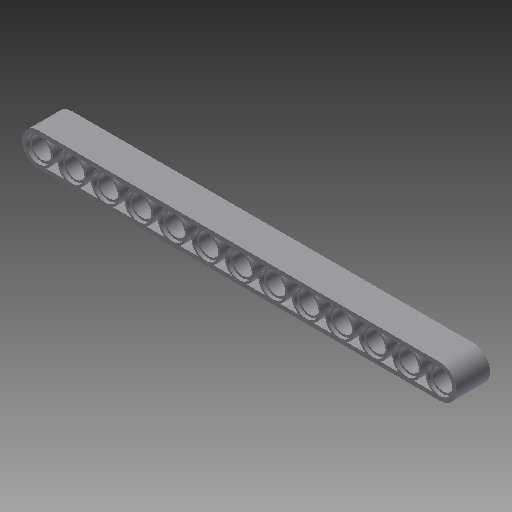
# Autodesk Inventor part: 13M Beam
Saved by Autodesk Inventor 2018 (Build 220112000, 112)
## iProperties
Created: 2014-02-10
Part Number: 13M Beam
Document SubType Name: Modeling
Designer: jleonard
Density: 1 g/cm^3
Material: Generic
Appearance: Default
Author: jleonard
Autodesk Inventor part; units mm, degrees
ref_plane "YZ Plane" through (0, 0, 0) normal (1, 0, 0) x (0, 1, 0)
ref_plane "XZ Plane" through (0, 0, 0) normal (0, 1, 0) x (-1, 0, 0)
ref_plane "XY Plane" through (0, 0, 0) normal (0, 0, 1) x (1, 0, 0)
sketch "Sketch2" plane through (0, 0, 0) normal (0, 0, 1) x (1, 0, 0)
  arc A0 (-48, 4) -> (-48, -4) centre (-48, 0) ccw
  arc A1 (48, -4) -> (48, 4) centre (48, 0) ccw
  line L0 (-48, 4) -> (48, 4)
  line L1 (-48, -4) -> (48, -4)
  line L2 (-72.8, 0) -> (72.8, 0) projected
  line L3 (0, -5.6) -> (0, 5.6) projected
  point P0 (0, 0)
  dimension "d0" = 4
  dimension "d1" = 4
  dimension "d2" = 96
  dimension "d3" = 0
  dimension "d4" = 48
  dimension "d9" = 180
  dimension "d10" = 0
  dimension "d225" = 96
  constraints: 6 point on circle, 4 end point, 2 centre point, 2 point on line, 2 tangent
  measures "d0" radius of A0
  measures "d1" radius of A1
  measures "d2" distance of A1.centre A0.centre
  measures "d3" distance from line of A0.centre L2
  measures "d4" distance from line of A0.centre L3
  measures "d9" angle of L0 L2
  measures "d10" distance from line of L2 A1.centre
  measures "d225" distance of L1.start L1.end
extrude "Extrusion1" add sketch "Sketch2" along normal blind 8
sketch "Sketch23" plane through (0, 0, 8) normal (0, 0, 1) x (1, 0, 0)
  arc A0 (-48, 4) -> (-48, -4) centre (-48, 0) ccw projected
  circle A1 centre (-48, 0) radius 2.5
  line L0 (-72.8, 0) -> (72.8, 0) projected
  circle A2 centre (-40, 0) radius 2.5
  circle A3 centre (-32, 0) radius 2.5
  circle A4 centre (-24, 0) radius 2.5
  circle A5 centre (-16, 0) radius 2.5
  circle A6 centre (-8, 0) radius 2.5
  circle A7 centre (0, 0) radius 2.5
  circle A8 centre (8, 0) radius 2.5
  circle A9 centre (16, 0) radius 2.5
  circle A10 centre (24, 0) radius 2.5
  circle A11 centre (32, 0) radius 2.5
  circle A12 centre (40, 0) radius 2.5
  circle A13 centre (48, 0) radius 2.5
  dimension "d226" = 5
  dimension "d232" = 8
  constraints: 13 centre point, 1 coincident, 1 horizontal, 24 other
  measures "d226" diameter of A1
  measures "d232" distance of A1.centre A2.centre
extrude "Extrusion22" cut sketch "Sketch23" against normal through all
sketch "Sketch24" plane through (0, 0, 8) normal (0, 0, 1) x (1, 0, 0)
  circle A0 centre (48, 0) radius 2.5 projected
  circle A1 centre (40, 0) radius 2.5 projected
  circle A2 centre (32, 0) radius 2.5 projected
  circle A3 centre (24, 0) radius 2.5 projected
  circle A4 centre (16, 0) radius 2.5 projected
  circle A5 centre (8, 0) radius 2.5 projected
  circle A6 centre (0, 0) radius 2.5 projected
  circle A7 centre (-8, 0) radius 2.5 projected
  circle A8 centre (-16, 0) radius 2.5 projected
  circle A9 centre (-24, 0) radius 2.5 projected
  circle A10 centre (-32, 0) radius 2.5 projected
  circle A11 centre (-40, 0) radius 2.5 projected
  circle A12 centre (-48, 0) radius 2.5 projected
  arc A13 (-48, 4) -> (-48, -4) centre (-48, 0) ccw projected
  circle A14 centre (-48, 0) radius 3
  line L0 (-72.8, 0) -> (72.8, 0) projected
  circle A15 centre (-40, 0) radius 3
  circle A16 centre (-32, 0) radius 3
  circle A17 centre (-24, 0) radius 3
  circle A18 centre (-16, 0) radius 3
  circle A19 centre (-8, 0) radius 3
  circle A20 centre (0, 0) radius 3
  circle A21 centre (8, 0) radius 3
  circle A22 centre (16, 0) radius 3
  circle A23 centre (24, 0) radius 3
  circle A24 centre (32, 0) radius 3
  circle A25 centre (40, 0) radius 3
  circle A26 centre (48, 0) radius 3
  dimension "d236" = 6
  dimension "d242" = 8
  constraints: 13 centre point, 1 coincident, 1 horizontal, 24 other
  measures "d236" diameter of A14
  measures "d242" distance of A14.centre A15.centre
extrude "Extrusion23" cut sketch "Sketch24" against normal blind 0.8 contours L0 A26 A0 | A0 L0 A26 | A14 L0 A12 | L0 A12 A14 | A15 L0 A11 | L0 A11 A15 | A16 L0 A10 | L0 A10 A16 | A17 L0 A9 | L0 A9 A17 | A18 L0 A8 | L0 A8 A18 | A19 L0 A7 | L0 A7 A19 | A20 L0 A6 | L0 A6 A20 | A21 L0 A5 | L0 A5 A21 | A22 L0 A4 | L0 A4 A22 | A23 L0 A3 | L0 A3 A23 | A24 L0 A2 | L0 A2 A24 | A25 L0 A1 | L0 A1 A25
sketch "Sketch25" plane through (0, 0, 0) normal (0, 0, -1) x (-1, 0, 0)
  circle A0 centre (-48, 0) radius 2.5 projected
  circle A1 centre (-40, 0) radius 2.5 projected
  circle A2 centre (-32, 0) radius 2.5 projected
  circle A3 centre (-24, 0) radius 2.5 projected
  circle A4 centre (-16, 0) radius 2.5 projected
  circle A5 centre (-8, 0) radius 2.5 projected
  circle A6 centre (0, 0) radius 2.5 projected
  circle A7 centre (8, 0) radius 2.5 projected
  circle A8 centre (16, 0) radius 2.5 projected
  circle A9 centre (24, 0) radius 2.5 projected
  circle A10 centre (32, 0) radius 2.5 projected
  circle A11 centre (40, 0) radius 2.5 projected
  circle A12 centre (48, 0) radius 2.5 projected
  arc A13 (-48, 4) -> (-48, -4) centre (-48, 0) ccw projected
  circle A14 centre (-48, 0) radius 3
  line L0 (72.8, 0) -> (-72.8, 0) projected
  circle A15 centre (-40, 0) radius 3
  circle A16 centre (-32, 0) radius 3
  circle A17 centre (-24, 0) radius 3
  circle A18 centre (-16, 0) radius 3
  circle A19 centre (-8, 0) radius 3
  circle A20 centre (0, 0) radius 3
  circle A21 centre (8, 0) radius 3
  circle A22 centre (16, 0) radius 3
  circle A23 centre (24, 0) radius 3
  circle A24 centre (32, 0) radius 3
  circle A25 centre (40, 0) radius 3
  circle A26 centre (48, 0) radius 3
  dimension "d246" = 6
  dimension "d252" = 8
  constraints: 13 centre point, 1 coincident, 1 horizontal, 24 other
  measures "d246" diameter of A14
  measures "d252" distance of A14.centre A15.centre
extrude "Extrusion24" cut sketch "Sketch25" against normal blind 0.8 contours L0 A14 A0 | A0 L0 A14 | A26 L0 A12 | L0 A12 A26 | A25 L0 A11 | L0 A11 A25 | A24 L0 A10 | L0 A10 A24 | A23 L0 A9 | L0 A9 A23 | A22 L0 A8 | L0 A8 A22 | A21 L0 A7 | L0 A7 A21 | A20 L0 A6 | L0 A6 A20 | A19 L0 A5 | L0 A5 A19 | A18 L0 A4 | L0 A4 A18 | A17 L0 A3 | L0 A3 A17 | A16 L0 A2 | L0 A2 A16 | A15 L0 A1 | L0 A1 A15
sketch "Sketch26" plane through (0, 0, 8) normal (0, 0, 1) x (1, 0, 0)
  circle A0 centre (-48, 0) radius 3 projected
  circle A1 centre (-40, 0) radius 3 projected
  arc A2 (-48, 4) -> (-48, -4) centre (-48, 0) ccw projected
  line L0 (-41.8028, -3) -> (-46.1972, -3)
  line L1 (-41.8028, 3) -> (-46.1972, 3)
  arc A3 (-41.8028, 3) -> (-41.8028, -3) centre (-40, 0) ccw
  arc A4 (-46.1972, -3) -> (-46.1972, 3) centre (-48, 0) ccw
  line L2 (-72.8, 0) -> (72.8, 0) projected
  line L3 (-33.8028, -3) -> (-38.1972, -3)
  line L4 (-33.8028, 3) -> (-38.1972, 3)
  arc A5 (-33.8028, 3) -> (-33.8028, -3) centre (-32, 0) ccw
  arc A6 (-38.1972, -3) -> (-38.1972, 3) centre (-40, 0) ccw
  line L5 (-25.8028, -3) -> (-30.1972, -3)
  line L6 (-25.8028, 3) -> (-30.1972, 3)
  arc A7 (-25.8028, 3) -> (-25.8028, -3) centre (-24, 0) ccw
  arc A8 (-30.1972, -3) -> (-30.1972, 3) centre (-32, 0) ccw
  line L7 (-17.8028, -3) -> (-22.1972, -3)
  line L8 (-17.8028, 3) -> (-22.1972, 3)
  arc A9 (-17.8028, 3) -> (-17.8028, -3) centre (-16, 0) ccw
  arc A10 (-22.1972, -3) -> (-22.1972, 3) centre (-24, 0) ccw
  line L9 (-9.8028, -3) -> (-14.1972, -3)
  line L10 (-9.8028, 3) -> (-14.1972, 3)
  arc A11 (-9.8028, 3) -> (-9.8028, -3) centre (-8, 0) ccw
  arc A12 (-14.1972, -3) -> (-14.1972, 3) centre (-16, 0) ccw
  line L11 (-1.8028, -3) -> (-6.1972, -3)
  line L12 (-1.8028, 3) -> (-6.1972, 3)
  arc A13 (-1.8028, 3) -> (-1.8028, -3) centre (0, 0) ccw
  arc A14 (-6.1972, -3) -> (-6.1972, 3) centre (-8, 0) ccw
  line L13 (6.1972, -3) -> (1.8028, -3)
  line L14 (6.1972, 3) -> (1.8028, 3)
  arc A15 (6.1972, 3) -> (6.1972, -3) centre (8, 0) ccw
  arc A16 (1.8028, -3) -> (1.8028, 3) centre (0, 0) ccw
  line L15 (14.1972, -3) -> (9.8028, -3)
  line L16 (14.1972, 3) -> (9.8028, 3)
  arc A17 (14.1972, 3) -> (14.1972, -3) centre (16, 0) ccw
  arc A18 (9.8028, -3) -> (9.8028, 3) centre (8, 0) ccw
  line L17 (22.1972, -3) -> (17.8028, -3)
  line L18 (22.1972, 3) -> (17.8028, 3)
  arc A19 (22.1972, 3) -> (22.1972, -3) centre (24, 0) ccw
  arc A20 (17.8028, -3) -> (17.8028, 3) centre (16, 0) ccw
  line L19 (30.1972, -3) -> (25.8028, -3)
  line L20 (30.1972, 3) -> (25.8028, 3)
  arc A21 (30.1972, 3) -> (30.1972, -3) centre (32, 0) ccw
  arc A22 (25.8028, -3) -> (25.8028, 3) centre (24, 0) ccw
  line L21 (38.1972, -3) -> (33.8028, -3)
  line L22 (38.1972, 3) -> (33.8028, 3)
  arc A23 (38.1972, 3) -> (38.1972, -3) centre (40, 0) ccw
  arc A24 (33.8028, -3) -> (33.8028, 3) centre (32, 0) ccw
  line L23 (46.1972, -3) -> (41.8028, -3)
  line L24 (46.1972, 3) -> (41.8028, 3)
  arc A25 (46.1972, 3) -> (46.1972, -3) centre (48, 0) ccw
  arc A26 (41.8028, -3) -> (41.8028, 3) centre (40, 0) ccw
  dimension "d257" = 7
  dimension "d258" = 7
  dimension "d264" = 8
  constraints: 48 end point, 48 point on circle, 24 centre point, 4 tangent, 2 coincident, 1 horizontal, 110 other
  measures "d257" diameter of A4
  measures "d258" diameter of A3
  measures "d264" distance of L1.start L4.start
extrude "Extrusion25" cut sketch "Sketch26" against normal through all contours A26 L24 A25 L2 | L2 A25 L23 A26 | A24 L22 A23 L2 | L2 A23 L21 A24 | A22 L20 A21 L2 | L2 A21 L19 A22 | A20 L18 A19 L2 | L2 A19 L17 A20 | A18 L16 A17 L2 | L2 A17 L15 A18 | A16 L14 A15 L2 | L2 A15 L13 A16 | A14 L12 A13 L2 | L2 A13 L11 A14 | A12 L10 A11 L2 | L2 A11 L9 A12 | A10 L8 A9 L2 | L2 A9 L7 A10 | A8 L6 A7 L2 | L2 A7 L5 A8 | A6 L4 A5 L2 | L2 A5 L3 A6 | A4 L1 A3 L2 | L2 A3 L0 A4
equation "\"d4\" = 0.5 * d2"
body "Solid1"
